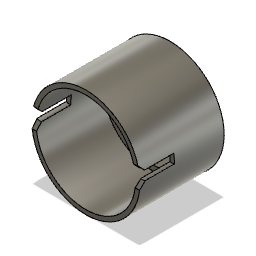
2ndSleeve_41mm (Autodesk Fusion 360 design; units mm, degrees)
Autodesk Fusion 360 part; units mm, degrees
sketch "Sketch1" plane through (0, 0, 0) normal (0, 0, 1) x (1, 0, 0)
  circle A0 centre (0, 0) radius 23
  circle A1 centre (0, 0) radius 25
  circle A2 centre (0, 0) radius 20.5
  dimension "d1" = 46
  dimension "d2" = 50
  dimension "d30" = 41
  constraint coincident A0.centre A1.centre
  constraint concentric A0 A1
  constraint concentric A1 A2
  measures "d1" diameter of A0
  measures "d2" diameter of A1
  measures "d30" diameter of A2
extrude "Extrude4" add sketch "Sketch1" along normal blind 5 contours A0 makes body 1
extrude "Extrude1" add sketch "Sketch1" along normal blind 39 separate body contours A0 | A1 | A2 makes body 2
extrude "Extrude2" add sketch "Sketch1" along normal blind 8 contours A1 bodies 2
hole "Hole1" at (23.8797, 1.871, 39) direction (0, 0, -1) diameter 4.5 depth 16 tip angle 180 countersink diameter 9.4 countersink angle 90 bodies 2
hole "Hole2" at (-23.5639, 1.6905, 39) direction (0, 0, -1) diameter 4.5 depth 16 tip angle 180 countersink diameter 9.4 countersink angle 90 bodies 2
hole "Hole3" at (0.0204, 7.1722, 39) direction (0, 0, -1) diameter 4.5 depth 16 tip angle 180 countersink diameter 9.4 countersink angle 90 bodies 2
hole "Hole4" at (0.0173, -8.1724, 39) direction (0, 0, -1) diameter 4.5 depth 16 tip angle 180 countersink diameter 9.4 countersink angle 90 bodies 2
extrude "Extrude3" cut sketch "Sketch1" along normal blind 60 contours A0 | A2 bodies 2
extrude "Extrude5" add 1 faces at (22.0047, -2.1611, 5) along direction (0, 0, 1) blind 3 on bodies 1 bodies 1 2
